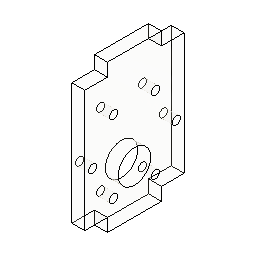
MotorDocking v5 (Autodesk Fusion 360 design; units mm, degrees)
Autodesk Fusion 360 part; units mm, degrees
sketch "Sketch1" plane through (0, 0, 0) normal (1, 0, 0) x (0, 1, 0)
  circle A0 centre (0, 0) radius 15.5 construction
  circle A1 centre (0, 15.5) radius 1.5 construction
  line L0 (0, 0) -> (0, 15.5) construction
  circle A2 centre (-13.4234, 7.75) radius 1.5 construction
  circle A3 centre (-13.4234, -7.75) radius 1.5 construction
  circle A4 centre (0, -15.5) radius 1.5 construction
  circle A5 centre (13.4234, -7.75) radius 1.5 construction
  circle A6 centre (13.4234, 7.75) radius 1.5 construction
  line L1 (0, 0) -> (-7, 0) construction
  circle A7 centre (-7, 0) radius 6 construction
  circle A8 centre (0, 0) radius 18.4 construction
  line L2 (-4.6, -1.8) -> (-4.6, 1.8) construction
  arc A9 (-4.6, 1.8) -> (-4.6, -1.8) centre (-7, 0) ccw construction
  dimension "d1" = 31
  dimension "d2" = 3
  dimension "d4" = 360
  dimension "d5" = 7
  dimension "d6" = 12
  dimension "d7" = 36.8
  dimension "d8" = 6
  dimension "d9" = 2.4
  constraint coincident A0.centre L0.start
  constraint coincident A0 A1.centre
  constraint vertical L0
  constraint coincident A1.centre L0.end
  constraint perpendicular L0 L1
  constraint coincident L1.end A7.centre
  constraint concentric A7 A9
  constraint perpendicular L1 L2
  measures "d1" diameter of A0
  measures "d2" diameter of A1
  measures "d5" distance of A0.centre L1.end
  measures "d6" diameter of A7
  measures "d7" diameter of A8
  measures "d8" diameter of A9
  measures "d9" distance of L1.end L2
sketch "Sketch2" plane through (0, 0, 0) normal (1, 0, 0) x (0, 1, 0)
  line L0 (-18.4, 18.4) -> (26.6, 18.4)
  line L1 (26.6, -18.4) -> (-18.4, -18.4)
  circle A0 centre (0, 0) radius 18.4
  circle A1 centre (-13.4234, 7.75) radius 1.5
  circle A2 centre (0, 15.5) radius 1.5
  circle A3 centre (13.4234, 7.75) radius 1.5
  circle A4 centre (13.4234, -7.75) radius 1.5
  circle A5 centre (0, -15.5) radius 1.5
  circle A6 centre (-13.4234, -7.75) radius 1.5
  circle A7 centre (-7, 0) radius 6
  line L2 (-18.4, 10) -> (-23.2, 10)
  line L3 (-23.2, 10) -> (-23.2, -10)
  line L4 (-23.2, -10) -> (-18.4, -10)
  line L5 (0, 0) -> (-23.2, 0) construction
  line L6 (-18.4, -18.4) -> (-18.4, -10)
  line L7 (-18.4, 10) -> (-18.4, 18.4)
  line L8 (26.6, 10) -> (31.4, 10)
  line L9 (31.4, 10) -> (31.4, -10)
  line L10 (31.4, -10) -> (26.6, -10)
  line L11 (0, 0) -> (31.4, 0) construction
  line L12 (26.6, 18.4) -> (26.6, 10)
  line L13 (26.6, -10) -> (26.6, -18.4)
  point P0 (-23.2, 0)
  point P1 (31.4, 0)
  dimension "d13" = 20
  dimension "d14" = 4.8
  dimension "d15" = 4.8
  dimension "d16" = 20
  dimension "d17" = 45
  constraint horizontal L0
  constraint vertical L12
  constraint horizontal L1
  constraint vertical L6
  constraint tangent A0 L6
  constraint tangent L0 A0
  constraint tangent L1 A0
  constraint coincident L2.start L6
  constraint perpendicular L2 L6
  constraint perpendicular L2 L3
  constraint perpendicular L4 L6
  constraint midpoint L3 P0
  constraint coincident A0.centre L5.start
  constraint coincident P0 L5.end
  constraint horizontal L5
  constraint collinear L6 L7
  constraint perpendicular L8 L12
  constraint perpendicular L8 L9
  constraint coincident L10.end L12
  constraint perpendicular L10 L12
  constraint midpoint L9 P1
  constraint coincident P1 L11.end
  constraint horizontal L11
  constraint collinear L12 L13
  measures "d13" distance of L2.end L3.end
  measures "d14" distance of L2.start L2.end
  measures "d15" distance of L8.start L8.end
  measures "d16" distance of L8.end L9.end
  measures "d17" distance of L0.start L0.end
extrude "Extrude1" add sketch "Sketch2" along normal blind 4.8
move_body "Move1" bodies 1 to x (1, 0, 0) y (0, 0, 1) z (0, -1, 0) at (0, -7, 7)
